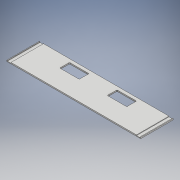
# Autodesk Inventor part: 뒷판
Saved by Autodesk Inventor 2017 (Build 210142000, 142)
## iProperties
Part Number: 뒷판
Material: 일반
Document SubType Name: Modeling
Designer: minom
Density: 1 g/cm^3
Appearance: 기본값
Author: minom
Autodesk Inventor part; units mm, degrees
ref_plane "YZ Plane" through (0, 0, 0) normal (1, 0, 0) x (0, 1, 0)
ref_plane "XZ Plane" through (0, 0, 0) normal (0, 1, 0) x (-1, 0, 0)
ref_plane "XY Plane" through (0, 0, 0) normal (0, 0, 1) x (1, 0, 0)
sketch "스케치1" plane through (0, 0, 0) normal (0, 0, 1) x (1, 0, 0)
  line L0 (90, -7) -> (-116, -7)
  line L1 (-116, -7) -> (-116, -57)
  line L2 (-116, -57) -> (90, -57)
  line L3 (90, -57) -> (90, -7)
  point P0 (0, 0)
  dimension "d0" = 50
  dimension "d3" = 206
  constraints: 8 end point, 2 parallel, 1 horizontal, 1 perpendicular
  measures "d0" distance of L1.end L0.end
  measures "d3" distance of L0.start L0.end
extrude "돌출1" add sketch "스케치1" along normal blind 2
sketch "스케치2" plane through (0, 0, 2) normal (0, 0, 1) x (1, 0, 0)
  line L0 (90, -7) -> (-116, -7) projected
  line L1 (-115, -7) -> (-109.6, -7)
  line L2 (-109.6, -7) -> (-109.6, -57.0095)
  line L3 (-109.6, -57.0095) -> (-115, -57.0095)
  line L4 (-115, -57.0095) -> (-115, -7)
  line L5 (-116, -7) -> (-116, -57) projected
  line L6 (-116, -57) -> (90, -57) projected
  line L7 (83.6, -7) -> (89, -7)
  line L8 (89, -7) -> (89, -57)
  line L9 (89, -57) -> (83.6, -57)
  line L10 (83.6, -57) -> (83.6, -7)
  line L11 (90, -57) -> (90, -7) projected
  point P0 (0, 0)
  dimension "d4" = 5.4
  dimension "d5" = 1
  dimension "d6" = 5.4
  dimension "d7" = 1
  constraints: 16 end point, 4 parallel, 3 point on line, 2 horizontal, 2 perpendicular
  measures "d4" distance of L2.end L3.end
  measures "d5" distance between parallel lines of L5 L4
  measures "d6" distance of L8.end L9.end
  measures "d7" distance between parallel lines of L11 L8
extrude "돌출2" cut sketch "스케치2" against normal blind 1 contours L8 L6 L10 L0 | L2 L6 L4 L0 | L2 L3 L4 L6
sketch "스케치3" plane through (0, 0, 2) normal (0, 0, 1) x (1, 0, 0)
  line L0 (83.6, -57) -> (83.6, -7) projected
  line L1 (83.6, -7) -> (-109.6, -7) projected
  line L2 (-109.6, -7) -> (-109.6, -57) projected
  line L3 (-109.6, -57) -> (83.6, -57) projected
  line L4 (-109.6, -29.3333) -> (-64.6, -29.3333)
  line L5 (83.6, -24) -> (38.6, -24)
  line L6 (90, -7) -> (-116, -7) projected
  line L7 (-13, -7) -> (-13, -12)
  line L8 (-13, -12) -> (-63.6, -12)
  line L9 (-109.6, -7) -> (-109.6, -57) projected
  line L10 (9.6, -12) -> (37.6, -12)
  line L11 (38.6, -26) -> (38.6, -13)
  line L12 (-64.6, -26) -> (-64.6, -13)
  line L13 (37.6, -12) -> (9.6, -12)
  line L14 (8.6, -13) -> (8.6, -26)
  line L15 (9.6, -27) -> (37.6, -27)
  line L16 (38.6, -26) -> (38.6, -13)
  line L17 (-63.6, -12) -> (-35.6, -12)
  line L18 (-34.6, -13) -> (-34.6, -26)
  line L19 (-35.6, -27) -> (-63.6, -27)
  line L20 (-64.6, -26) -> (-64.6, -13)
  arc A0 (-34.6, -13) -> (-35.6, -12) centre (-35.6, -13) ccw
  arc A1 (-35.6, -27) -> (-34.6, -26) centre (-35.6, -26) ccw
  arc A2 (-64.6, -26) -> (-63.6, -27) centre (-63.6, -26) ccw
  arc A3 (-63.6, -12) -> (-64.6, -13) centre (-63.6, -13) ccw
  arc A4 (9.6, -12) -> (8.6, -13) centre (9.6, -13) ccw
  arc A5 (38.6, -13) -> (37.6, -12) centre (37.6, -13) ccw
  arc A6 (37.6, -27) -> (38.6, -26) centre (37.6, -26) ccw
  arc A7 (8.6, -26) -> (9.6, -27) centre (9.6, -26) ccw
  point P0 (0, 0)
  point P1 (83.6, -12)
  point P2 (38.6, -12)
  point P3 (-64.6, -12)
  point P4 (8.6, -27)
  point P5 (8.6, -12)
  point P6 (38.6, -27)
  point P7 (-34.6, -27)
  point P8 (-34.6, -12)
  point P9 (-64.6, -27)
  dimension "d10" = 45
  dimension "d11" = 45
  dimension "d12" = 5
  dimension "d13" = 30
  dimension "d14" = 15
  dimension "d15" = 30
  dimension "d16" = 15
  dimension "d19" = 1
  constraints: 30 end point, 22 point on line, 16 point on circle, 16 tangent, 8 centre point, 7 equal radius, 5 perpendicular, 4 horizontal, 4 parallel, 1 midpoint, 1 vertical
  measures "d10" distance of L4.start L4.end
  measures "d11" distance of L5.start L5.end
  measures "d12" distance of L7.start L7.end
  measures "d13" distance of point (38.6, -27) point (8.6, -27)
  measures "d14" distance of point (8.6, -27) point (8.6, -12)
  measures "d15" distance of point (-34.6, -27) point (-64.6, -27)
  measures "d16" distance of point (-34.6, -12) point (-34.6, -27)
  measures "d19" radius of A0
extrude "돌출3" cut sketch "스케치3" against normal blind 10 contours A0 L18 A1 L19 A2 L12 A3 L8 | L10 A5 L11 A6 L15 A7 L14 A4
